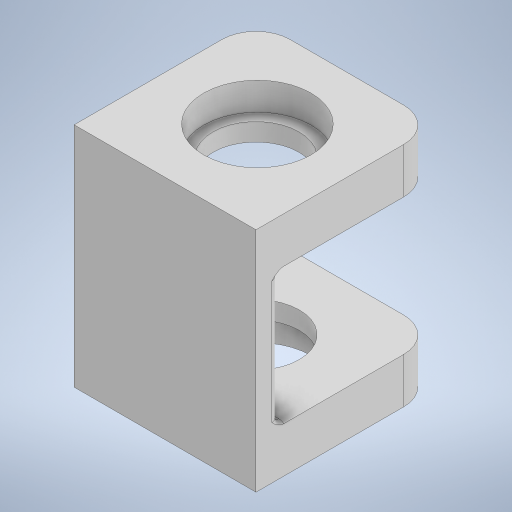
# Autodesk Inventor part: ApoioBaseCilindrica47_5
Saved by Autodesk Inventor 2023.2 (Build 272271030, 271C)
## iProperties
Created: 2023-04-15
Part Number: ApoioBaseCilindrica47_5
Material: Generic
Document SubType Name: Modeling
Designer: victo
Density: 1 g/cm^3
Appearance: Default
Author: victo
## iProperties of the stored document ApoioBaseCilindrica47_5_3DPrint.ipt
Created: 2023-05-06
Part Number: ApoioBaseCilindrica47_5_3DPrint
Material: Generic
Document SubType Name: Modeling
Designer: victo
Density: 1 g/cm^3
Appearance: Default
Author: victo
Autodesk Inventor part; units mm, degrees
ref_plane "YZ Plane" through (0, 0, 0) normal (1, 0, 0) x (0, 1, 0)
ref_plane "XZ Plane" through (0, 0, 0) normal (0, 1, 0) x (-1, 0, 0)
ref_plane "XY Plane" through (0, 0, 0) normal (0, 0, 1) x (1, 0, 0)
sketch "Sketch1" plane through (0, 0, 0) normal (0, 1, 0) x (-1, 0, 0)
  line L0 (-40, 40) -> (40, 40)
  line L1 (40, 40) -> (40, -40)
  line L2 (40, -40) -> (-40, -40)
  line L3 (-40, -40) -> (-40, 40)
  line L4 (-40, 40) -> (40, -40) construction
  line L5 (40, 40) -> (-40, -40) construction
  point P0 (0, 0)
  dimension "d11" = 80
  dimension "d12" = 80
  constraints: 12 end point, 2 midpoint, 2 parallel, 1 horizontal, 1 perpendicular
  measures "d11" distance of L0.end L1.end
  measures "d12" distance of L1.end L2.end
extrude "Extrusion1" add sketch "Sketch1" along normal blind 20
sketch "Sketch2" plane through (0, 20, 0) normal (0, 1, 0) x (1, 0, 0)
  line L0 (40, 40) -> (-40, 40) projected
  line L1 (-40, 40) -> (-40, -40) projected
  line L2 (-40, -40) -> (40, -40) projected
  line L3 (40, -40) -> (40, 40) projected
  line L4 (-40, -40) -> (40, -40)
  line L5 (40, -40) -> (40, -30)
  line L6 (40, -30) -> (-40, -30)
  line L7 (-40, -30) -> (-40, -40)
  point P0 (0, 0)
  dimension "d2" = 10
  constraints: 8 end point, 2 parallel, 1 horizontal, 1 perpendicular, 1 point on line
  measures "d2" distance of L5.end L4.end
extrude "Extrusion2" add sketch "Sketch2" along normal blind 80 contours L3 L2 L1 L6
sketch "Sketch7" plane through (0, 20, 0) normal (0, 1, 0) x (1, 0, 0)
  line L0 (-40, -30) -> (40, -30) projected
  line L1 (40, -30) -> (40, 40) projected
  line L2 (40, 40) -> (-40, 40) projected
  line L3 (-40, 40) -> (-40, -30) projected
  arc A0 (-40, -30) -> (-40, -30) centre (0, 7.8333) ccw projected
  point P0 (0, 0)
  constraints: 1 other
sketch "Sketch8" plane through (40, 20, 30) normal (0, 0, -1) x (-1, 0, 0)
  line L0 (0, -20) -> (0, 80) projected
  line L1 (80, -20) -> (80, 80) projected
  line L2 (0, 80) -> (80, 80)
  line L3 (80, 80) -> (80, 60)
  line L4 (80, 60) -> (0, 60)
  line L5 (0, 60) -> (0, 80)
  point P0 (40, -20)
  point P1 (80, 80)
  dimension "d16" = 20
  constraints: 8 end point, 2 parallel, 1 horizontal, 1 perpendicular, 1 point on line
  measures "d16" distance of L2.end L3.end
extrude "Extrusion6" add sketch "Sketch8" along normal blind 70
fillet "Fillet1" radius 15 4 edges at (40, 90, -40) (-40, 90, -40) (-40, 10, -40) (40, 10, -40)
fillet "Fillet2" radius 3 4 edges at (0, 80, 30) (0, 20, 30) (-40, 50, 30) (40, 50, 30)
sketch "Sketch17" plane through (0, 100, 0) normal (0, 1, 0) x (1, 0, 0)
  arc A0 (-25, 40) -> (-40, 25) centre (-25, 25) ccw projected
  line L0 (-40, -40) -> (-40, 25) projected
  line L1 (-40, -40) -> (40, -40) projected
  line L2 (40, -40) -> (40, 25) projected
  arc A1 (40, 25) -> (25, 40) centre (25, 25) ccw projected
  line L3 (-25, 40) -> (25, 40) projected
  line L4 (-40, -40) -> (40, -40) projected
  line L5 (0, -40) -> (0, -23)
  circle A2 centre (0, 0.6) radius 23.6
  point P0 (0, 0)
  dimension "d57" = 47.2
  dimension "d56" = 17
  constraints: 2 end point, 1 midpoint, 1 vertical, 1 vertical alignment, 2 other
  measures "d56" distance of L5.start L5.end
extrude "Extrusion15" cut sketch "Sketch17" against normal blind 110 contours A2
sketch "Sketch19" plane through (-25, 80, -40) normal (0, -1, 0) x (1, 0, 0)
  circle A0 centre (25, 40) radius 19
  circle A1 centre (25, 39.4) radius 23.6 projected
  circle A2 centre (25, 39.4) radius 23.6 projected
  dimension "d63" = 38
  constraints: 1 centre point, 1 coincident
  measures "d63" diameter of A0
extrude "Extrusion17" add sketch "Sketch19" against normal blind 7.8
sketch "Sketch20" plane through (0, 20, 0) normal (0, 1, 0) x (1, 0, 0)
  circle A0 centre (0, 0) radius 19
  circle A1 centre (0, 0.6) radius 23.6 projected
  dimension "d66" = 38
  constraints: 1 centre point, 1 coincident
  measures "d66" diameter of A0
extrude "Extrusion18" add sketch "Sketch20" against normal blind 7.8
body "Solid1"
